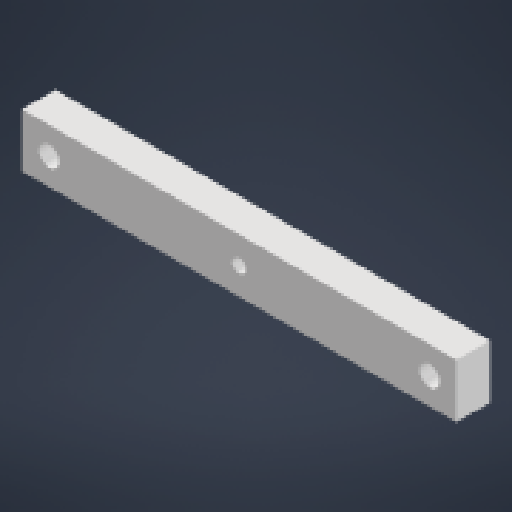
# Autodesk Inventor part: vertical_axis_hal_holder
Saved by Autodesk Inventor 2023.2 (Build 272271000, 271)
## iProperties
Created: 2023-07-30
Part Number: vertical_axis_hal_holder
Material: Generic
Document SubType Name: Modeling
Designer: Bober
Density: 1 g/cm^3
Appearance: Default
Author: Bober
Autodesk Inventor part; units mm, degrees
ref_plane "YZ Plane" through (0, 0, 0) normal (1, 0, 0) x (0, 1, 0)
ref_plane "XZ Plane" through (0, 0, 0) normal (0, 1, 0) x (-1, 0, 0)
ref_plane "XY Plane" through (0, 0, 0) normal (0, 0, 1) x (1, 0, 0)
sketch "Sketch1" plane through (0, 0, 0) normal (0, 0, 1) x (1, 0, 0)
  circle A0 centre (-56.5936, 0) radius 1.5 projected
  line L0 (-52.5936, 4) -> (-60.5936, 4) projected
  line L1 (-60.5936, 4) -> (-60.5936, -4) projected
  line L2 (-60.5936, -4) -> (-52.5936, -4) projected
  line L3 (-52.5936, -4) -> (-52.5936, 4) projected
  circle A1 centre (0, 0) radius 1.5 projected
  line L4 (-4, 4) -> (-4, -4) projected
  line L5 (-4, -4) -> (4, -4) projected
  line L6 (4, -4) -> (4, 4) projected
  line L7 (4, 4) -> (-4, 4) projected
  line L8 (-60.5936, 4) -> (4, 4)
  line L9 (4, 4) -> (4, -4)
  line L10 (4, -4) -> (-60.5936, -4)
  line L11 (-60.5936, -4) -> (-60.5936, 4)
  point P0 (0, 0)
  constraints: 8 end point, 2 parallel, 1 horizontal, 1 perpendicular
extrude "Extrusion1" add sketch "Sketch1" along normal blind 5
sketch "Sketch2" plane through (0, 0, 0) normal (0, 0, -1) x (-1, 0, 0)
  point P0 (0, 0)
sketch "Sketch3" plane through (0, 0, 0) normal (0, 0, -1) x (-1, 0, 0)
  line L0 (60.5936, 4) -> (60.5936, -4) projected
  line L1 (-4, 4) -> (60.5936, 4) projected
  line L2 (-4, -4) -> (-4, 4) projected
  line L3 (60.5936, -4) -> (-4, -4) projected
  circle A0 centre (0, 0) radius 1.5 projected
  circle A1 centre (56.5936, 0) radius 1.5 projected
  circle A2 centre (28.2966, 0) radius 1.95
  point P0 (0, 0)
  point P1 (60.5936, 0)
  dimension "d2" = 3.9
  dimension "d4" = 32.297
  constraints: 1 centre point, 1 horizontal alignment, 1 midpoint
  measures "d2" diameter of A2
  measures "d4" distance from line of L0 A2.centre
extrude "Extrusion2" cut sketch "Sketch3" against normal blind 1.8 contours A2
sketch "Sketch4" plane through (-28.2966, 0, 1.8) normal (0, 0, -1) x (-1, 0, 0)
  circle A0 centre (0, 0) radius 1
  point P0 (-28.2966, 0)
  dimension "d7" = 2
  constraints: 1 centre point
  measures "d7" diameter of A0
extrude "Extrusion3" cut sketch "Sketch4" against normal through all
body "Solid1"
